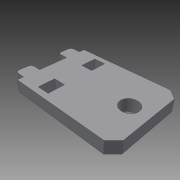
# Autodesk Inventor part: y_carriage_belt_iddler
Saved by Autodesk Inventor 2014 (Build 180170000, 170)
## iProperties
Created: 2013-11-29
Part Number: y_carriage_belt_iddler
Material: Generic
Document SubType Name: Modeling
Designer: buben
Density: 1 g/cm^3
Appearance: Anodized - Dark Gray
Author: buben
Subject: Laser Cutted
Autodesk Inventor part; units mm, degrees
ref_plane "YZ Plane" through (0, 0, 0) normal (1, 0, 0) x (0, 1, 0)
ref_plane "XZ Plane" through (0, 0, 0) normal (0, 1, 0) x (-1, 0, 0)
ref_plane "XY Plane" through (0, 0, 0) normal (0, 0, 1) x (1, 0, 0)
sketch "Sketch1" plane through (0, 0, 0) normal (0, 0, 1) x (1, 0, 0)
  line L0 (0, 0) -> (47, 0)
  line L1 (51, 4) -> (51, 33)
  line L2 (47, 37) -> (0, 37)
  line L3 (0, 37) -> (0, 0)
  circle A0 centre (42, 18.5) radius 4.25
  line L4 (47, 37) -> (51, 33)
  line L5 (47, 0) -> (51, 4)
  line L6 (10, 34) -> (16, 34)
  line L7 (16, 34) -> (16, 26)
  line L8 (16, 26) -> (10, 26)
  line L9 (10, 26) -> (10, 34)
  line L10 (10, 11) -> (16, 11)
  line L11 (16, 11) -> (16, 3)
  line L12 (16, 3) -> (10, 3)
  line L13 (10, 3) -> (10, 11)
  line L14 (10, 26) -> (16, 11) construction
  line L15 (10, 11) -> (16, 26) construction
  circle A1 centre (42, 18.5) radius 16 construction
  line L16 (24, 37) -> (24, 0) construction
  point P0 (51, 37)
  point P1 (51, 0)
  point P2 (0, 18.5)
  point P3 (13, 18.5)
  dimension "d0" = 4
  dimension "d1" = 4
  dimension "d2" = 4
  dimension "d3" = 4
  dimension "d4" = 8.5
  dimension "d5" = 37
  dimension "d6" = 6
  dimension "d7" = 8
  dimension "d8" = 8
  dimension "d9" = 15
  dimension "d10" = 10
  dimension "d11" = 32
  dimension "d12" = 9
  dimension "d13" = 26
  dimension "d14" = 24
  constraints: 34 end point, 6 parallel, 6 point on line, 4 perpendicular, 3 horizontal, 2 centre point, 2 collinear, 2 horizontal alignment, 2 midpoint, 1 coincident
  measures "d0" distance of L2.start point (51, 37)
  measures "d1" distance of L1.end point (51, 37)
  measures "d2" distance of L0.end point (51, 0)
  measures "d3" distance of L1.start point (51, 0)
  measures "d4" diameter of A0
  measures "d5" distance of L2.end L0.start
  measures "d6" distance of L6.start L6.end
  measures "d7" distance of L8.end L6.start
  measures "d8" distance of L12.end L10.start
  measures "d9" distance between parallel lines of L8 L10
  measures "d10" distance between parallel lines of L3 L9
  measures "d11" diameter of A1
  measures "d12" distance from line of L1 A0.centre
  measures "d13" distance from line of L7 A0.centre
  measures "d14" distance between parallel lines of L3 L16
extrude "Extrusion1" add sketch "Sketch1" along normal blind 6
sketch "Sketch2" plane through (0, 0, 6) normal (0, 0, 1) x (1, 0, 0)
  line L0 (16, 26) -> (10, 26) projected
  line L1 (0, 37) -> (0, 0) projected
  line L2 (0, 34) -> (-4, 34)
  line L3 (-6, 32) -> (-6, 28)
  line L4 (-4, 26) -> (0, 26)
  line L5 (0, 26) -> (0, 34)
  line L6 (0, 11) -> (-4, 11)
  line L7 (-6, 9) -> (-6, 5)
  line L8 (-4, 3) -> (0, 3)
  line L9 (0, 3) -> (0, 11)
  arc A0 (-4, 34) -> (-6, 32) centre (-4, 32) ccw
  arc A1 (-6, 28) -> (-4, 26) centre (-4, 28) ccw
  arc A2 (-4, 11) -> (-6, 9) centre (-4, 9) ccw
  arc A3 (-6, 5) -> (-4, 3) centre (-4, 5) ccw
  dimension "d17" = 2
  dimension "d18" = 6
  dimension "d19" = 8
  dimension "d20" = 8
  dimension "d21" = 15
  constraints: 16 end point, 8 point on circle, 8 tangent, 4 centre point, 4 parallel, 3 equal radius, 2 collinear, 2 horizontal, 2 perpendicular, 2 point on line
  measures "d17" radius of A0
  measures "d18" distance between parallel lines of L1 L3
  measures "d19" distance between parallel lines of L4 L2
  measures "d20" distance between parallel lines of L8 L6
  measures "d21" distance between parallel lines of L6 L4
extrude "Extrusion2" add sketch "Sketch2" against normal blind 6
equation "\"d1\" = d0"
equation "\"d2\" = d0"
equation "\"d3\" = d2"
body "Solid1"
